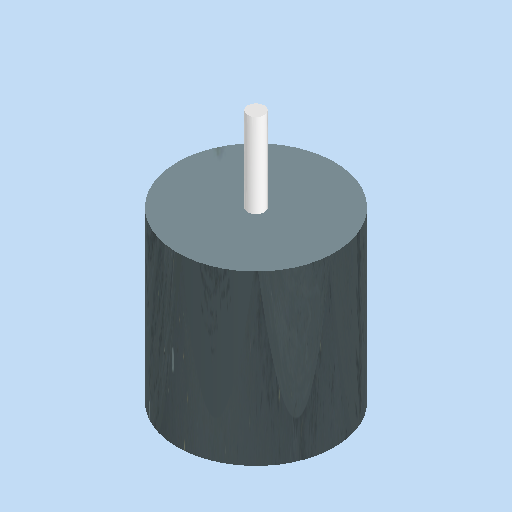
# Autodesk Inventor part: 电机
Saved by Autodesk Inventor 2026.2 (Build 302298010, 298A)
## iProperties
Created: 2026-03-16
Part Number: 电机
Material: 常规
Document SubType Name: Modeling
Designer: liu
Density: 1 g/cm^3
Appearance: 默认
Author: liu
Autodesk Inventor part; units mm, degrees
ref_plane "YZ Plane" through (0, 0, 0) normal (1, 0, 0) x (0, 1, 0)
ref_plane "XZ Plane" through (0, 0, 0) normal (0, 1, 0) x (-1, 0, 0)
ref_plane "XY Plane" through (0, 0, 0) normal (0, 0, 1) x (1, 0, 0)
sketch "草图1" plane through (0, 0, 0) normal (0, 1, 0) x (-1, 0, 0)
  circle A0 centre (7.9754, 4.9539) radius 14
  point P0 (0, 0)
  dimension "d0" = 28
  constraints: 1 centre point
  measures "d0" diameter of A0
extrude "拉伸1" add sketch "草图1" along normal blind 30
sketch "草图2" plane through (-7.9754, 30, 4.9539) normal (0, 1, 0) x (1, 0, 0)
  circle A0 centre (0, 0) radius 1.5
  point P0 (7.9754, 4.9539)
  dimension "d3" = 3
  constraints: 1 centre point
  measures "d3" diameter of A0
extrude "拉伸2" add sketch "草图2" along normal blind 15
